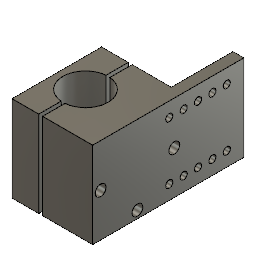
Motor EMT Mount (Autodesk Fusion 360 design; units mm, degrees)
Autodesk Fusion 360 part; units mm, degrees
note: some values were not read from the file. Set by a fixed rule: which face or edge a step refers to.
sketch "Sketch1" plane through (0, 0, 0) normal (0, 1, 0) x (1, 0, 0)
  line L0 (-1, -11.75) -> (-1, -17.6498)
  line L1 (1, -11.75) -> (1, -17.75)
  line L2 (-1, -11.75) -> (-1, -11.7074)
  line L3 (1, -11.75) -> (1, -11.7074)
  arc A0 (1, -11.7074) -> (-1, -11.7074) centre (0, 0) ccw
  line L4 (-1, -17.6498) -> (-1, -17.8661)
  line L5 (1, -17.75) -> (1, -17.8661)
  line L6 (10, -11.8998) -> (-10, -11.8998)
  line L7 (-10, -11.8998) -> (-10, -23.8998)
  line L8 (-10, -23.8998) -> (10, -23.8998)
  line L9 (10, -23.8998) -> (10, -11.8998)
  line L10 (10, -11.8998) -> (-10, -23.8998) construction
  line L11 (-10, -11.8998) -> (10, -23.8998) construction
  line L12 (-1, -17.6498) -> (-1, -23.8998)
  line L13 (1, -17.75) -> (1, -23.8998)
  line L14 (15, -15) -> (-15, -15)
  line L15 (-15, -15) -> (-15, 15)
  line L16 (-15, 15) -> (15, 15)
  line L17 (15, 15) -> (15, -15)
  line L18 (15, -15) -> (-15, 15) construction
  line L19 (-15, -15) -> (15, 15) construction
  line L20 (-1, -17.6498) -> (-1, -17.8661)
  line L21 (1, -17.75) -> (1, -23.8998)
  line L22 (-10, -11.8998) -> (10, -23.8998) construction
  line L23 (10, -11.8998) -> (-10, -23.8998) construction
  line L24 (-1, -17.6498) -> (-1, -23.8998)
  line L25 (1, -11.75) -> (1, -17.75)
  line L26 (-10, -11.8998) -> (-10, -23.8998)
  line L27 (1, -17.75) -> (1, -17.8661)
  line L28 (-1, -11.75) -> (-1, -17.6498)
  line L29 (10, -11.8998) -> (-10, -11.8998)
  line L30 (1, -11.75) -> (1, -11.7074)
  line L31 (-10, -23.8998) -> (10, -23.8998)
  line L32 (10, -23.8998) -> (10, -11.8998)
  line L33 (-1, -11.75) -> (-1, -11.7074)
  line L34 (1, 24.25) -> (1, 18.25)
  line L35 (1, 18.25) -> (1, 18.1339)
  line L36 (-10, 24.1002) -> (10, 12.1002) construction
  line L37 (-1, 18.3502) -> (-1, 12.1002)
  line L38 (10, 12.1002) -> (10, 24.1002)
  line L39 (-1, 24.25) -> (-1, 24.2926)
  line L40 (1, 24.25) -> (1, 18.25)
  line L41 (-1, 24.25) -> (-1, 24.2926)
  line L42 (-1, 18.3502) -> (-1, 18.1339)
  line L43 (10, 12.1002) -> (10, 24.1002)
  line L44 (-1, 18.3502) -> (-1, 18.1339)
  line L45 (1, 18.25) -> (1, 12.1002)
  line L46 (-10, 24.1002) -> (-10, 12.1002)
  line L47 (-10, 12.1002) -> (10, 12.1002)
  line L48 (-1, 24.25) -> (-1, 18.3502)
  line L49 (10, 24.1002) -> (-10, 12.1002) construction
  line L50 (1, 24.25) -> (1, 24.2926)
  line L51 (-10, 24.1002) -> (-10, 12.1002)
  line L52 (10, 24.1002) -> (-10, 12.1002) construction
  line L53 (-1, 24.25) -> (-1, 18.3502)
  line L54 (10, 24.1002) -> (-10, 24.1002)
  line L55 (10, 24.1002) -> (-10, 24.1002)
  line L56 (-10, 12.1002) -> (10, 12.1002)
  line L57 (-1, 18.3502) -> (-1, 12.1002)
  line L58 (1, 18.25) -> (1, 18.1339)
  line L59 (1, 24.25) -> (1, 24.2926)
  line L60 (-10, 24.1002) -> (10, 12.1002) construction
  line L61 (1, 18.25) -> (1, 12.1002)
  line L62 (-1, 12.1002) -> (-1, 11.7074)
  line L63 (1, 12.1002) -> (1, 11.7074)
  line L64 (10, -23.8998) -> (15, -23.8998)
  line L65 (15, -23.8998) -> (15, -15)
  line L66 (15, -15) -> (10, -15)
  line L67 (10, -15) -> (10, -23.8998)
  line L68 (-10, -23.8998) -> (-15, -23.8998)
  line L69 (-15, -23.8998) -> (-15, -15)
  line L70 (-15, -15) -> (-10, -15)
  line L71 (-10, -15) -> (-10, -23.8998)
  line L72 (-10, 24.1002) -> (-15, 24.1002)
  line L73 (-15, 24.1002) -> (-15, 15)
  line L74 (-15, 15) -> (-10, 15)
  line L75 (-10, 15) -> (-10, 24.1002)
  line L76 (10, 24.1002) -> (15, 24.1002)
  line L77 (15, 24.1002) -> (15, 15)
  line L78 (15, 15) -> (10, 15)
  line L79 (10, 15) -> (10, 24.1002)
  point P0 (0, -17.8998)
  point P1 (0, -17.8998)
  point P2 (0, 18.1002)
  point P3 (0, 18.1002)
  dimension "d1" = 23.5
  dimension "d15" = 20
  dimension "d16" = 12
  dimension "d33" = 30
  dimension "d34" = 30
  dimension "d86" = 20
  dimension "d87" = 12
  dimension "d88" = 20
  dimension "d89" = 12
  dimension "d90" = 20
  dimension "d91" = 12
  constraint coincident A0.centre origin
  constraint parallel L0 L2
  constraint parallel L1 L3
  constraint parallel L0 L4
  constraint vertical L5
  constraint horizontal L6
  constraint perpendicular L6 L7
  constraint parallel L6 L8
  constraint parallel L7 L9
  constraint coincident L10 P1
  constraint coincident L11 P1
  constraint coincident L8 L12.end
  constraint perpendicular L8 L12
  constraint coincident L8 L13.end
  constraint perpendicular L8 L13
  constraint horizontal L14
  constraint perpendicular L14 L15
  constraint parallel L14 L16
  constraint parallel L15 L17
  constraint coincident L18 A0.centre
  constraint coincident L19 A0.centre
  constraint parallel L28 L33
  constraint parallel L25 L30
  constraint parallel L20 L28
  constraint vertical L27
  constraint horizontal L29
  constraint perpendicular L26 L29
  constraint parallel L29 L31
  constraint parallel L26 L32
  constraint coincident P1 L23
  constraint coincident P1 L22
  constraint coincident L12.end L31
  constraint perpendicular L24 L31
  constraint coincident L13.end L31
  constraint perpendicular L21 L31
  constraint parallel L39 L48
  constraint parallel L34 L50
  constraint parallel L44 L48
  constraint vertical L35
  constraint horizontal L54
  constraint perpendicular L51 L54
  constraint parallel L47 L54
  constraint parallel L43 L51
  constraint coincident P3 L52
  constraint coincident P3 L36
  constraint coincident L37.end L47
  constraint perpendicular L37 L47
  constraint coincident L45.end L47
  constraint perpendicular L45 L47
  constraint parallel L41 L53
  constraint parallel L40 L59
  constraint parallel L42 L53
  constraint vertical L58
  constraint horizontal L55
  constraint perpendicular L46 L55
  constraint parallel L55 L56
  constraint parallel L38 L46
  constraint coincident P3 L49
  constraint coincident P3 L60
  constraint coincident L37.end L56
  constraint perpendicular L56 L57
  constraint coincident L45.end L56
  constraint perpendicular L56 L61
  constraint coincident A0 L62.end
  constraint perpendicular L47 L62
  constraint coincident A0 L63.end
  constraint perpendicular L56 L63
  constraint horizontal L64
  constraint vertical L65
  constraint horizontal L66
  constraint vertical L67
  constraint horizontal L68
  constraint vertical L69
  constraint horizontal L70
  constraint vertical L71
  constraint horizontal L72
  constraint vertical L73
  constraint horizontal L74
  constraint vertical L75
  constraint horizontal L76
  constraint vertical L77
  constraint horizontal L78
  constraint vertical L79
  measures "d1" diameter of A0
  measures "d15" distance of L7.end L8.end
  measures "d16" distance of L6.end L7.end
  measures "d33" distance of L15.end L16.end
  measures "d34" distance of L14.end L15.end
  measures "d86" distance of L7.end L8.end
  measures "d87" distance of L6.end L7.end
  measures "d88" distance of L46.end L36.end
  measures "d89" distance of L36.start L46.end
  measures "d90" distance of L46.end L36.end
  measures "d91" distance of L36.start L46.end
extrude "Extrude1" add sketch "Sketch1" along normal blind 40 contours L0 L2 A0 L6 L7 L14 L15 L16 L26 L28 L29 L33 L46 L47 L51 L56 L62 L70 L74 | L0 L6 L7 L14 L26 L28 L29 | L1 L6 L9 L14 L25 L29 L32 | L1 L3 A0 L6 L9 L14 L16 L17 L25 L29 L30 L32 L38 L43 L47 L56 L63 L66 L78 | L16 L37 L46 L47 L51 L56 L57 | L16 L38 L43 L45 L47 L56 L61 makes body 1 at (-10.3385, 26.6667, -5.5836) makes body 2 at (6.9217, 26.6667, -9.4948)
extrude "Extrude2" add sketch "Sketch1" along normal blind 9.235 from surface at 15.3825 contours L0 L4 L7 L8 L12 L14 L20 L24 L26 L28 L31 L71 | L1 L5 L8 L9 L13 L14 L21 L25 L27 L31 L32 L67 | L7 L14 L26 L68 L69 L70 L71 | L9 L14 L32 L64 L65 L66 L67 | L16 L37 L42 L44 L46 L48 L51 L53 L54 L55 L57 L75 | L16 L46 L51 L72 L73 L74 L75 | L16 L34 L35 L38 L40 L43 L45 L54 L55 L58 L61 L79 | L16 L38 L43 L76 L77 L78 L79 bodies 1 2
ref_plane "WorkPlane2" through (27.1, 0, 0) normal (1, 0, 0) x (0, 1, 0)
sketch "Sketch8" plane through (27.1, 0, 0) normal (1, 0, 0) x (0, 0, -1)
  line L0 (-15, 0) -> (15, 0)
  line L1 (15, 0) -> (15, 40)
  line L2 (15, 40) -> (-15, 40)
  line L3 (-15, 40) -> (-15, 0)
  circle A0 centre (16.6, 5) radius 1.85
  circle A1 centre (16.6, 35) radius 1.85
  line L4 (-23.4, 42.5) -> (-23.4, -2.5)
  line L5 (-23.4, 42.5) -> (26.6, 42.5)
  line L6 (26.6, -2.5) -> (-23.4, -2.5)
  line L7 (-23.4, -2.5) -> (-23.4, 42.5)
  circle A2 centre (24.1, 5) radius 1.85
  circle A3 centre (46.6, 5) radius 1.85
  circle A4 centre (39.1, 35) radius 1.85
  line L8 (55.6, -2.5) -> (14.1, -2.5)
  circle A5 centre (31.6, 5) radius 1.85
  circle A6 centre (24.1, 35) radius 1.85
  circle A7 centre (31.6, 35) radius 1.85
  circle A8 centre (46.6, 35) radius 1.85
  circle A9 centre (39.1, 5) radius 1.85
  line L9 (14.1, 42.5) -> (55.6, 42.5)
  line L10 (46.6, 35) -> (48.45, 35)
  line L11 (46.6, 35) -> (55.6, 35)
  line L12 (14.1, -2.5) -> (14.1, 0)
  line L13 (14.1, 40) -> (14.1, 42.5)
  line L14 (14.1, 42.5) -> (14.1, 40)
  line L15 (14.1, 0) -> (14.1, -2.5)
  line L16 (6.6, 42.5) -> (6.6, -2.5)
  line L17 (46.6, 35) -> (55.6, 35)
  line L18 (55.6, 35) -> (55.6, 42.5)
  line L19 (55.6, 35) -> (55.6, -2.5)
  dimension "d62" = 3.7
  dimension "d63" = 3.7
  dimension "d105" = 50
  dimension "d106" = 45
  dimension "d107" = 3.7
  dimension "d108" = 3.7
  dimension "d111" = 3.7
  dimension "d112" = 3.7
  dimension "d113" = 3.7
  dimension "d114" = 3.7
  dimension "d115" = 3.7
  dimension "d116" = 3.7
  dimension "d118" = 45
  dimension "d149" = 9
  constraint vertical L4
  constraint horizontal L5
  constraint horizontal L6
  constraint vertical L7
  constraint vertical L14
  constraint horizontal L9
  constraint horizontal L8
  constraint vertical L12
  constraint coincident A8.centre L10.start
  constraint parallel L9 L10
  constraint coincident A8 L10.end
  constraint coincident L0 L12.end
  constraint coincident L2 L13.start
  constraint collinear L12 L13
  constraint collinear L14 L15
  constraint coincident L5 L16.start
  constraint coincident L6 L16.end
  constraint perpendicular L6 L16
  constraint parallel L11 L17
  constraint perpendicular L17 L18
  constraint perpendicular L11 L19
  measures "d62" diameter of A0
  measures "d63" diameter of A1
  measures "d105" distance of L4.start L5.end
  measures "d106" distance of L4.start L4.end
  measures "d107" diameter of A2
  measures "d108" diameter of A6
  measures "d111" diameter of A4
  measures "d112" diameter of A9
  measures "d113" diameter of A5
  measures "d114" diameter of A3
  measures "d115" diameter of A7
  measures "d116" diameter of A8
  measures "d118" distance of L9.start L8.end
  measures "d149" distance of A8.centre L11.end
extrude "Extrude22" add sketch "Sketch8" against normal blind 5.75 separate body contours L0 L1 L2 A0 A1 L16 | L0 L6 L12 L15 L16 | L0 L1 L2 A0 A1 L5 L6 L8 L9 L12 L13 L14 L15 L18 L19 | L0 L2 L3 L4 L5 L6 L7 L16 | L0 L2 L3 L16 | L2 L5 L13 L14 L16 makes body 3
extrude "Extrude23" add 1 faces at (15, 29.745, -5) along direction (1, 0, 0) up to surface (6.35 mm away) on bodies 2 bodies 2 3
sketch "Sketch10" plane through (-15, 0, 0) normal (-1, 0, 0) x (0, 0, 1)
  line L0 (-15, 0) -> (15, 0)
  line L1 (15, 0) -> (15, 15.3825)
  line L2 (15, 15.3825) -> (23.8998, 15.3825)
  line L3 (23.8998, 15.3825) -> (23.8998, 24.6175)
  line L4 (23.8998, 24.6175) -> (15, 24.6175)
  line L5 (15, 24.6175) -> (15, 40)
  line L6 (15, 40) -> (-15, 40)
  line L7 (-15, 40) -> (-15, 24.6175)
  line L8 (-15, 24.6175) -> (-24.1002, 24.6175)
  line L9 (-24.1002, 24.6175) -> (-24.1002, 15.3825)
  line L10 (-24.1002, 15.3825) -> (-15, 15.3825)
  line L11 (-15, 15.3825) -> (-15, 0)
  line L12 (23.4, 24.6175) -> (23.4, 42.5)
  line L13 (15, 24.6175) -> (23.4, 24.6175)
  line L14 (-15, 24.6175) -> (-23.4, 24.6175)
  line L15 (-23.4, 24.6175) -> (-23.4, 15.3825)
  line L16 (-23.4, 15.3825) -> (-15, 15.3825)
  line L17 (-15, 15.3825) -> (-15, 24.6175)
  line L18 (15, 24.6175) -> (23.4, 24.6175)
  line L19 (23.4, 24.6175) -> (23.4, 15.3825)
  line L20 (23.4, 15.3825) -> (15, 15.3825)
  line L21 (15, 15.3825) -> (15, 24.6175)
  dimension "d129" = 8.4
  dimension "d130" = 8.4
  constraint coincident L4.end L5.start
  constraint coincident L12.start L13.end
  constraint horizontal L14
  constraint vertical L15
  constraint horizontal L16
  constraint vertical L17
  constraint coincident L7.end L8.start
  constraint horizontal L18
  constraint vertical L19
  constraint horizontal L20
  constraint vertical L21
  measures "d129" distance of L7.end L14.end
  measures "d130" distance of L4.end L12.start
extrude "Extrude24" cut sketch "Sketch10" against normal up to surface (36.35 mm away) contours L8 L9 L10 L15 | L2 L3 L4 L19 bodies 1 2
sketch "Sketch11" plane through (-15, 0, 0) normal (-1, 0, 0) x (0, 0, 1)
  line L0 (-23.4, 24.6175) -> (-23.4, 15.3825)
  line L1 (-23.4, 15.3825) -> (-15, 15.3825)
  line L2 (-15, 15.3825) -> (-15, 0)
  line L3 (-15, 0) -> (15, 0)
  line L4 (15, 0) -> (15, 15.3825)
  line L5 (15, 15.3825) -> (23.4, 15.3825)
  line L6 (23.4, 15.3825) -> (23.4, 24.6175)
  line L7 (23.4, 24.6175) -> (15, 24.6175)
  line L8 (15, 24.6175) -> (15, 40)
  line L9 (15, 40) -> (-15, 40)
  line L10 (-15, 40) -> (-15, 24.6175)
  line L11 (-15, 24.6175) -> (-23.4, 24.6175)
  line L12 (-23.4, 15.3825) -> (-19.2, 20)
  circle A0 centre (-19.2, 20) radius 1.5
  line L13 (23.4, 15.3825) -> (19.2, 20)
  circle A1 centre (19.2, 20) radius 1.5
  line L14 (-21.95, 18.4123) -> (-19.2, 16.8246)
  line L15 (-19.2, 16.8246) -> (-16.45, 18.4123)
  line L16 (-16.45, 18.4123) -> (-16.45, 21.5877)
  line L17 (-16.45, 21.5877) -> (-19.2, 23.1754)
  line L18 (-19.2, 23.1754) -> (-21.95, 21.5877)
  line L19 (-21.95, 21.5877) -> (-21.95, 18.4123)
  line L20 (21.95, 21.5877) -> (19.2, 23.1754)
  line L21 (19.2, 23.1754) -> (16.45, 21.5877)
  line L22 (16.45, 21.5877) -> (16.45, 18.4123)
  line L23 (16.45, 18.4123) -> (19.2, 16.8246)
  line L24 (19.2, 16.8246) -> (21.95, 18.4123)
  line L25 (21.95, 18.4123) -> (21.95, 21.5877)
  point P0 (-19.2, 20)
  point P1 (19.2, 20)
  dimension "d133" = 3
  dimension "d134" = 3
  dimension "d135" = 2.75
  dimension "d136" = 2.75
  constraint coincident L0.end L1.start
  constraint coincident P0 L12.end
  constraint coincident L5.end L6.start
  constraint coincident P1 L13.end
  measures "d133" diameter of A0
  measures "d134" diameter of A1
  measures "d135" distance of P0 L19
  measures "d136" distance of P1 L25
extrude "Extrude25" cut sketch "Sketch11" against normal up to surface (42.1 mm away) contours A0 | A1 bodies 1 2
extrude "Extrude26" cut sketch "Sketch11" against normal blind 3.9 contours L14 L15 L16 L17 L18 L19 | L20 L21 L22 L23 L24 L25 bodies 1
sketch "Sketch12" plane through (27.1, 0, 0) normal (1, 0, 0) x (0, 0, -1)
  circle A0 centre (-19.2, 20) radius 1.5
  circle A1 centre (19.2, 20) radius 1.5
  circle A2 centre (24.1, 5) radius 1.85
  circle A3 centre (16.6, 35) radius 1.85
  circle A4 centre (46.6, 35) radius 1.85
  circle A5 centre (39.1, 35) radius 1.85
  circle A6 centre (39.1, 5) radius 1.85
  circle A7 centre (46.6, 5) radius 1.85
  circle A8 centre (16.6, 5) radius 1.85
  circle A9 centre (31.6, 5) radius 1.85
  circle A10 centre (31.6, 35) radius 1.85
  circle A11 centre (24.1, 35) radius 1.85
  line L0 (55.6, 42.5) -> (-23.4, 42.5)
  line L1 (-23.4, 42.5) -> (-23.4, -2.5)
  line L2 (-23.4, -2.5) -> (55.6, -2.5)
  circle A12 centre (-19.2, 20) radius 2.825
  circle A13 centre (19.2, 20) radius 2.825
  line L3 (55.6, -2.5) -> (55.6, 42.5)
  dimension "d141" = 5.65
  dimension "d142" = 5.65
  constraint concentric A0 A12
  constraint concentric A1 A13
  measures "d141" diameter of A12
  measures "d142" diameter of A13
extrude "Extrude27" cut sketch "Sketch12" against normal blind 17.1 contours A12 | A13 bodies 2
extrude "Extrude28" add 2 faces at (18.15, 0, 0) (-6.7946, 0, 13.6339) along direction (0, -1, 0) up to surface end surface through (27.1, -2.5, -14.1) normal (0, -1, 0) offset 0 on bodies 1 2 bodies 2 1
extrude "Extrude29" add 2 faces at (18.15, 40, 0) (-6.7946, 40, 13.6339) along direction (0, 1, 0) up to surface end surface through (27.1, 42.5, -26.6) normal (0, 1, 0) offset 0 on bodies 1 2 bodies 2 1
extrude "Extrude30" add 2 faces at (21.35, 3.4608, 17.8) (21.35, 30.5783, 20.6) along direction (-1, 0, 0) blind 20.35 on bodies 2 bodies 2
sketch "Sketch13" plane through (21.35, 0, 0) normal (-1, 0, 0) x (0, 0, 1)
  line L0 (-15, 35.9287) -> (-15, 42.5)
  line L1 (-15, 42.5) -> (-55.6, 42.5)
  line L2 (-55.6, 42.5) -> (-55.6, -2.5)
  line L3 (-55.6, -2.5) -> (-15, -2.5)
  line L4 (-15, -2.5) -> (-15, 4.0713)
  arc A0 (-15, 5.9287) -> (-15, 4.0713) centre (-16.6, 5) ccw
  line L5 (-15, 5.9287) -> (-15, 15.3825)
  line L6 (-15, 15.3825) -> (-23.4, 15.3825)
  line L7 (-23.4, 15.3825) -> (-23.4, 24.6175)
  line L8 (-23.4, 24.6175) -> (-15, 24.6175)
  line L9 (-15, 24.6175) -> (-15, 34.0713)
  arc A1 (-15, 35.9287) -> (-15, 34.0713) centre (-16.6, 35) ccw
  circle A2 centre (-24.1, 5) radius 1.85
  circle A3 centre (-46.6, 5) radius 1.85
  circle A4 centre (-46.6, 35) radius 1.85
  circle A5 centre (-31.6, 35) radius 1.85
  circle A6 centre (-24.1, 35) radius 1.85
  circle A7 centre (-39.1, 35) radius 1.85
  circle A8 centre (-31.6, 5) radius 1.85
  circle A9 centre (-39.1, 5) radius 1.85
  line L10 (-23.4, 24.6175) -> (-15, 24.6175)
  line L11 (-15, 24.6175) -> (-15, 42.5)
  line L12 (-15, 42.5) -> (-23.4, 42.5)
  line L13 (-23.4, 42.5) -> (-23.4, 24.6175)
  line L14 (-23.4, 15.3825) -> (-15, 15.3825)
  line L15 (-15, 15.3825) -> (-15, -2.5)
  line L16 (-15, -2.5) -> (-23.4, -2.5)
  line L17 (-23.4, -2.5) -> (-23.4, 15.3825)
  constraint horizontal L10
  constraint vertical L11
  constraint horizontal L12
  constraint vertical L13
  constraint coincident L0.end L1.start
  constraint coincident L7.end L8.start
  constraint horizontal L14
  constraint vertical L15
  constraint horizontal L16
  constraint vertical L17
  constraint coincident L3.end L4.start
  constraint coincident L6.end L7.start
extrude "Extrude31" add sketch "Sketch13" along normal blind 20.35 contours L0 L1 L8 L9 A1 A6 L10 L11 L12 L13 | A1 L11 | A6 L13 | L3 L4 A0 L5 L6 A2 L14 L15 L16 L17 | A2 L17 | A0 L15 picked at (-22.899, 35.4992) picked at (-22.8872, 4.9131) bodies 2
extrude "Extrude32" add 2 faces at (-10.3333, 30.5783, -15) (-5.6667, 9.4217, -15) along direction (0, 0, -1) blind 8.4 on bodies 1 bodies 1
extrude "Extrude33" add 2 faces at (-5.6667, 3.4608, 15) (-5.6667, 30.5783, 15) along direction (0, 0, 1) blind 8.4 on bodies 1 bodies 1
sketch "Sketch14" plane through (27.1, 0, 0) normal (1, 0, 0) x (0, 0, -1)
  circle A0 centre (-19.2, 20) radius 2.825
  circle A1 centre (19.2, 20) radius 2.825
  circle A2 centre (24.1, 5) radius 1.85
  circle A3 centre (46.6, 5) radius 1.85
  circle A4 centre (16.6, 5) radius 1.85
  circle A5 centre (46.6, 35) radius 1.85
  circle A6 centre (16.6, 35) radius 1.85
  circle A7 centre (31.6, 35) radius 1.85
  circle A8 centre (24.1, 35) radius 1.85
  circle A9 centre (39.1, 35) radius 1.85
  circle A10 centre (31.6, 5) radius 1.85
  circle A11 centre (39.1, 5) radius 1.85
  line L0 (55.6, -2.5) -> (55.6, 42.5)
  line L1 (55.6, 42.5) -> (-23.4, 42.5)
  line L2 (-23.4, 42.5) -> (-23.4, -2.5)
  line L3 (-23.4, -2.5) -> (55.6, -2.5)
  line L4 (-23.4, -2.5) -> (0, -2.5)
  line L5 (0, -2.5) -> (0, 1.5)
  line L6 (-1.5877, 4.25) -> (-3.1754, 1.5)
  line L7 (-3.1754, 1.5) -> (-1.5877, -1.25)
  line L8 (1.5877, 4.25) -> (-1.5877, 4.25)
  line L9 (1.5877, -1.25) -> (3.1754, 1.5)
  line L10 (-1.5877, -1.25) -> (1.5877, -1.25)
  circle A12 centre (0, 1.5) radius 1.5
  line L11 (3.1754, 1.5) -> (1.5877, 4.25)
  circle A13 centre (0, 1.5) radius 2.8
  point P0 (0, 1.5)
  point P1 (0, 1.5)
  dimension "d158" = 23.4
  dimension "d159" = 4
  dimension "d161" = 3
  dimension "d162" = 2.75
  dimension "d168" = 5.6
  constraint coincident L2.end L3.start
  constraint perpendicular L2 L4
  constraint perpendicular L3 L5
  constraint coincident P1 P0
  measures "d158" distance of L2.end L4.end
  measures "d159" distance of L4.end P1
  measures "d161" diameter of A12
  measures "d162" distance of P1 L7
  measures "d168" diameter of A13
extrude "Extrude34" cut sketch "Sketch14" against normal blind 20 contours A12 bodies 2
extrude "Extrude35" cut sketch "Sketch14" along normal blind 7 from surface at -20 contours L6 L7 L8 L9 L10 L11 A13 | L7 L10 A13 | L9 L10 A13 | L6 L7 A13 | L9 L11 A13 | L6 L8 A13 | L8 L11 A13 bodies 2
extrude "Extrude36" cut sketch "Sketch14" against normal blind 7 contours L5 L10 A13 | L5 L10 A13 | L6 L7 L8 L9 L10 L11 A13 | L7 A13 | L9 A13 | L11 A13 | L8 A13 bodies 2
equation "d135 = ( 5.5 / 2 ) * 1 mm"
equation "d136 = ( 5.5 / 2 ) * 1 mm"
equation "d143 = -3.2 mm - 13.9 mm"
equation "d158 = ( 46.8 / 2 ) * 1 mm"
equation "d162 = ( 5.5 / 2 ) * 1 mm"
